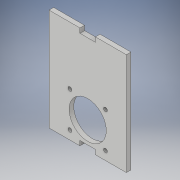
# Autodesk Inventor part: side_plate
Saved by Autodesk Inventor 2017 (Build 210142000, 142)
## iProperties
Created: 2017-06-15
Part Number: side_plate
Material: Generic
Document SubType Name: Modeling
Designer: millerid
Density: 1 g/cm^3
Appearance: Default
Author: millerid
Autodesk Inventor part; units mm, degrees
ref_plane "YZ Plane" through (0, 0, 0) normal (1, 0, 0) x (0, 1, 0)
ref_plane "XZ Plane" through (0, 0, 0) normal (0, 1, 0) x (-1, 0, 0)
ref_plane "XY Plane" through (0, 0, 0) normal (0, 0, 1) x (1, 0, 0)
sketch "Sketch1" plane through (0, 0, 0) normal (0, 0, 1) x (1, 0, 0)
  line L0 (50, 0) -> (50, 60)
  line L1 (0, 60) -> (0, 0)
  line L2 (20, 0) -> (20, -3)
  line L3 (20, -3) -> (0, -3)
  line L4 (0, -3) -> (0, 0)
  line L5 (30, 0) -> (30, -3)
  line L6 (30, -3) -> (50, -3)
  line L7 (50, -3) -> (50, 0)
  line L8 (20, 0) -> (30, 0)
  line L9 (20, 60) -> (20, 63)
  line L10 (20, 63) -> (0, 63)
  line L11 (0, 63) -> (0, 60)
  line L12 (30, 60) -> (30, 63)
  line L13 (30, 63) -> (50, 63)
  line L14 (50, 63) -> (50, 60)
  line L15 (30, 60) -> (20, 60)
  circle A0 centre (25, 14) radius 12
  circle A1 centre (13.5, 2.6) radius 1.25
  circle A2 centre (36.5, 2.6) radius 1.25
  circle A3 centre (13.5, 25.6) radius 1.25
  circle A4 centre (36.5, 25.6) radius 1.25
  point P0 (25, 0)
  dimension "d0" = 50
  dimension "d1" = 60
  dimension "d2" = 20
  dimension "d3" = 3
  dimension "d4" = 20
  dimension "d5" = 20
  dimension "d6" = 3
  dimension "d7" = 20
  dimension "d8" = 24
  dimension "d9" = 14
  dimension "d10" = 25
  dimension "d11" = 2.5
  dimension "d12" = 2.6
  dimension "d13" = 11.5
  dimension "d14" = 2.5
  dimension "d15" = 11.5
  dimension "d16" = 2.5
  dimension "d17" = 23
  dimension "d18" = 2.5
  constraints: 32 end point, 5 centre point, 5 parallel, 2 horizontal, 2 point on line, 1 midpoint
  measures "d0" distance of L1.start L0.end
  measures "d1" distance of L0.end L0.start
  measures "d2" distance of L2.end L3.end
  measures "d3" distance of L2.start L2.end
  measures "d4" distance of L6.end L5.end
  measures "d5" distance of L10.end L9.end
  measures "d6" distance of L9.end L9.start
  measures "d7" distance of L12.end L13.end
  measures "d8" diameter of A0
  measures "d9" distance from line of A0.centre L8
  measures "d10" distance from line of L0 A0.centre
  measures "d11" diameter of A1
  measures "d12" distance from line of L8 A1.centre
  measures "d13" horizontal distance of A1.centre point (25, 0)
  measures "d14" diameter of A2
  measures "d15" horizontal distance of A2.centre point (25, 0)
  measures "d16" diameter of A3
  measures "d17" distance of A1.centre A3.centre
  measures "d18" diameter of A4
extrude "Extrusion1" add sketch "Sketch1" along normal blind 3
equation "\"d15\" = d13"
body "Solid1"
